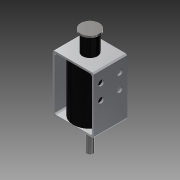
# Autodesk Inventor part: Solenoid
Saved by Autodesk Inventor 2015 (Build 190159000, 159)
## iProperties
Created: 2016-09-21
Part Number: Solenoid
Material: Generic
Document SubType Name: Modeling
Designer: James Yelland
Density: 1 g/cm^3
Appearance: Default
Author: James Yelland
Autodesk Inventor part; units mm, degrees
ref_plane "YZ Plane" through (0, 0, 0) normal (1, 0, 0) x (0, 1, 0)
ref_plane "XZ Plane" through (0, 0, 0) normal (0, 1, 0) x (-1, 0, 0)
ref_plane "XY Plane" through (0, 0, 0) normal (0, 0, 1) x (1, 0, 0)
sketch "Sketch1" plane through (0, 0, 0) normal (0, 1, 0) x (-1, 0, 0)
  line L0 (-11, 14.2) -> (-11, -14.2)
  line L1 (-10, -15.2) -> (10, -15.2)
  line L2 (11, -14.2) -> (11, 14.2)
  line L3 (10, 15.2) -> (-10, 15.2)
  line L4 (-11, 15.2) -> (11, -15.2) construction
  line L5 (-11, -15.2) -> (11, 15.2) construction
  line L6 (-10, 13.2) -> (-10, -13.2)
  line L7 (-9, -14.2) -> (9, -14.2)
  line L8 (10, -13.2) -> (10, 13.2)
  line L9 (9, 14.2) -> (-9, 14.2)
  line L10 (-10, 14.2) -> (10, -14.2) construction
  line L11 (-10, -14.2) -> (10, 14.2) construction
  arc A0 (11, 14.2) -> (10, 15.2) centre (10, 14.2) ccw
  arc A1 (10, 13.2) -> (9, 14.2) centre (9, 13.2) ccw
  arc A2 (9, -14.2) -> (10, -13.2) centre (9, -13.2) ccw
  arc A3 (10, -15.2) -> (11, -14.2) centre (10, -14.2) ccw
  arc A4 (-10, -13.2) -> (-9, -14.2) centre (-9, -13.2) ccw
  arc A5 (-11, -14.2) -> (-10, -15.2) centre (-10, -14.2) ccw
  arc A6 (-10, 15.2) -> (-11, 14.2) centre (-10, 14.2) ccw
  arc A7 (-9, 14.2) -> (-10, 13.2) centre (-9, 13.2) ccw
  point P0 (0, 0)
  dimension "d0" = 30.4
  dimension "d1" = 22
  dimension "d2" = 28.4
  dimension "d3" = 20
  dimension "d4" = 1
  dimension "d5" = 1
  constraints: 24 end point, 16 point on circle, 16 point on line, 16 tangent, 8 centre point, 6 equal radius, 4 midpoint, 4 parallel, 2 perpendicular, 2 vertical
  measures "d0" distance of L4.start L5.start
  measures "d1" distance of L4.end L5.start
  measures "d2" distance of L10.start L11.start
  measures "d3" distance of L10.end L11.start
  measures "d4" radius of A0
  measures "d5" radius of A4
extrude "Extrusion1" add sketch "Sketch1" along normal blind 18
sketch "Sketch3" plane through (-9, 0, -14.2) normal (0, 0, 1) x (1, 0, 0)
  line L0 (9, 0) -> (9, 9)
  circle A0 centre (9, 9) radius 9
  dimension "d12" = 9
  dimension "d13" = 18
  constraints: 2 end point, 1 centre point, 1 coincident, 1 vertical
  measures "d12" distance of L0.start L0.end
  measures "d13" diameter of A0
extrude "Extrusion3" add sketch "Sketch3" along normal up to surface (28.4 mm away)
sketch "Sketch4" plane through (-10, 0, 15.2) normal (0, 0, 1) x (1, 0, 0)
  circle A0 centre (10, 9) radius 4
  point P0 (10, 0)
  dimension "d16" = 8
  constraints: 1 centre point
  measures "d16" diameter of A0
extrude "Extrusion4" add sketch "Sketch4" along normal blind 10
sketch "Sketch5" plane through (0, 9, 25.2) normal (0, 0, 1) x (1, 0, 0)
  circle A0 centre (0, 0) radius 5
  point P0 (0, -9)
  dimension "d19" = 10
  constraints: 1 centre point
  measures "d19" diameter of A0
extrude "Extrusion5" add sketch "Sketch5" along normal blind 1
sketch "Sketch7" plane through (10, 0, -15.2) normal (0, 0, -1) x (-1, 0, 0)
  line L0 (10, 9) -> (10, 0)
  circle A0 centre (10, 9) radius 1.75
  dimension "d22" = 3.5
  constraints: 2 end point, 1 centre point, 1 coincident, 1 vertical
  measures "d22" diameter of A0
extrude "Extrusion6" add sketch "Sketch7" along normal blind 16
sketch "Sketch8" plane through (11, 0, 14.2) normal (1, 0, 0) x (0, 0, -1)
  line L0 (-1, 0) -> (-1, 18) projected
  line L1 (-1, 9) -> (5.5, 9)
  line L2 (5.5, 9) -> (5.5, 14)
  line L3 (5.5, 14) -> (5.5, 4)
  line L4 (5.5, 4) -> (13.5, 4)
  line L5 (13.5, 4) -> (13.5, 14)
  circle A0 centre (5.5, 14) radius 1.5
  circle A1 centre (13.5, 14) radius 1.5
  circle A2 centre (13.5, 4) radius 1.5
  circle A3 centre (5.5, 4) radius 1.5
  point P0 (14.2, 0)
  dimension "d25" = 6.5
  dimension "d26" = 5
  dimension "d27" = 10
  dimension "d28" = 8
  dimension "d29" = 3
  dimension "d30" = 3
  dimension "d31" = 3
  dimension "d32" = 3
  constraints: 10 end point, 4 centre point, 4 coincident, 3 perpendicular, 1 horizontal, 1 midpoint, 1 point on line
  measures "d25" distance of L1.start L1.end
  measures "d26" distance of L1.end L2.end
  measures "d27" distance of L2.end L3.end
  measures "d28" distance of L3.end L4.end
  measures "d29" diameter of A0
  measures "d30" diameter of A1
  measures "d31" diameter of A2
  measures "d32" diameter of A3
extrude "Extrusion7" cut sketch "Sketch8" against normal blind 2
body "Solid1"
